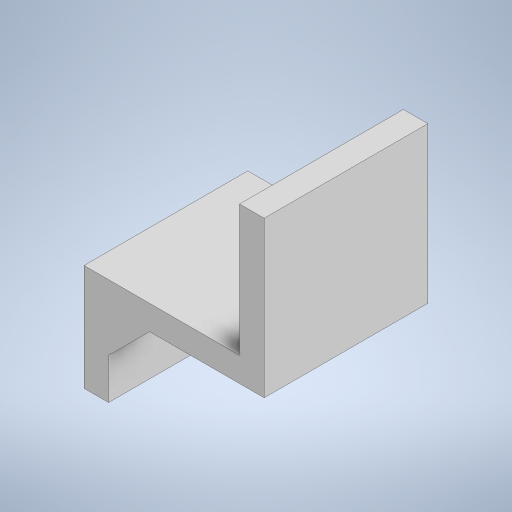
# Autodesk Inventor part: LED strip mount v02
Saved by Autodesk Inventor 2023 (Build 270158000, 158)
## iProperties
Created: 2024-06-26
Part Number: LED strip mount v02
Material: Generic
Document SubType Name: Modeling
Designer: Akramilab
Density: 1 g/cm^3
Appearance: Default
Author: Akramilab
Autodesk Inventor part; units mm, degrees
ref_plane "YZ Plane" through (0, 0, 0) normal (1, 0, 0) x (0, 1, 0)
ref_plane "XZ Plane" through (0, 0, 0) normal (0, 1, 0) x (-1, 0, 0)
ref_plane "XY Plane" through (0, 0, 0) normal (0, 0, 1) x (1, 0, 0)
sketch "Sketch1" plane through (0, 0, 0) normal (0, 0, 1) x (1, 0, 0)
  line L0 (0, 0) -> (22, 0)
  line L1 (22, 0) -> (22, -19)
  line L2 (22, -19) -> (0, -19)
  line L3 (0, -19) -> (0, 0)
  line L4 (3, 0) -> (19, 0)
  line L5 (19, 0) -> (19, -16)
  line L6 (19, -16) -> (3, -16)
  line L7 (3, -16) -> (3, 0)
  dimension "d0" = 22
  dimension "d1" = 19
  dimension "d2" = 3
  dimension "d3" = 3
  dimension "d4" = 3
  constraints: 16 end point, 4 parallel, 2 horizontal, 2 perpendicular, 1 point on line
  measures "d0" distance between parallel lines of L1 L3
  measures "d1" distance between parallel lines of L2 L0
  measures "d2" distance between parallel lines of L7 L3
  measures "d3" distance between parallel lines of L2 L6
  measures "d4" distance between parallel lines of L5 L1
extrude "Extrusion1" add sketch "Sketch1" along normal blind 20 contours L0 L7 L6 L5 L1 L2 L3
sketch "Sketch4" plane through (3, -16, 0) normal (1, 0, 0) x (0, 0, -1)
  line L0 (-20, 0) -> (-20, 16) projected
  line L1 (0, 0) -> (-20, 0)
  line L2 (-20, 0) -> (-20, 16)
  line L3 (-20, 16) -> (0, 16)
  line L4 (0, 16) -> (0, 0)
  constraints: 8 end point, 2 parallel, 1 horizontal, 1 perpendicular
extrude "Extrusion4" cut sketch "Sketch4" against normal through all
sketch "Sketch5" plane through (0, 0, 0) normal (0, 0, -1) x (-1, 0, 0)
  line L0 (0, -19) -> (-22, -19) projected
  line L1 (0, -19) -> (-3, -19)
  line L2 (-3, -19) -> (-3, -29)
  line L3 (-3, -29) -> (0, -29)
  line L4 (0, -29) -> (0, -19)
  point P0 (0, 0)
  dimension "d17" = 3
  dimension "d18" = 10
  constraints: 8 end point, 2 parallel, 1 horizontal, 1 perpendicular
  measures "d17" distance of L3.end L2.end
  measures "d18" distance of L2.end L1.end
extrude "Extrusion5" add sketch "Sketch5" against normal blind 20
sketch "Sketch6" plane through (3, -29, 0) normal (1, 0, 0) x (0, 0, -1)
  line L0 (0, 10) -> (-20, 10) projected
  line L1 (0, 10) -> (0, 0) projected
  circle A0 centre (-10, 5) radius 2.5
  point P0 (0, 29)
  dimension "d21" = 5
  dimension "d22" = 10
  dimension "d23" = 5
  constraints: 1 centre point, 1 coincident
  measures "d21" distance from line of point (-10, 5) L0
  measures "d22" distance from line of L1 point (-10, 5)
  measures "d23" diameter of A0
extrude "Extrusion6" cut sketch "Sketch6" against normal through all
sketch "Sketch7" plane through (0, 0, 0) normal (0, 0, -1) x (-1, 0, 0)
  line L0 (-3, -19) -> (-22, -19) projected
  line L1 (-3, -29) -> (-3, -19) projected
  line L2 (-8, -19) -> (-3, -24)
  point P0 (0, 0)
  dimension "d26" = 5
  dimension "d27" = 5
  constraints: 2 end point, 1 midpoint, 1 point on line
  measures "d26" distance of L0.start L2.start
  measures "d27" distance of L2.end L0.start
extrude "Extrusion7" add sketch "Sketch7" against normal blind 4
sketch "Sketch8" plane through (0, 0, 20) normal (0, 0, 1) x (1, 0, 0)
  line L0 (3, -19) -> (22, -19) projected
  line L1 (3, -29) -> (3, -19) projected
  line L2 (8, -19) -> (3, -24)
  point P0 (0, 0)
  dimension "d30" = 5
  dimension "d31" = 5
  constraints: 2 end point, 1 midpoint, 1 point on line
  measures "d30" distance of L2.start L0.start
  measures "d31" distance of L2.end L0.start
extrude "Extrusion8" add sketch "Sketch8" against normal blind 4
equation "\"d3\" = d2"
equation "\"d4\" = d2"
equation "\"d27\" = d26"
equation "\"d30\" = d26"
equation "\"d31\" = d30"
body "Solid1"
